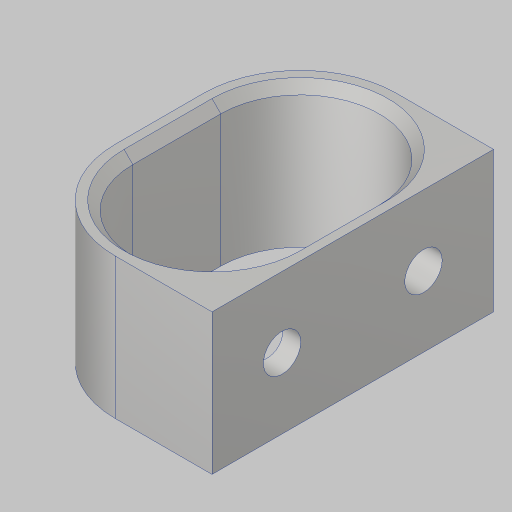
# Autodesk Inventor part: WL-007
Saved by Autodesk Inventor 2023.5 (Build 275446000, 446)
## iProperties
Created: 2025-02-28
Part Number: WL-007
Material: Aluminum 6061
Document SubType Name: Modeling
Designer: slick
Density: 2.7 g/cm^3
Appearance: Aluminum - Flat
Author: slick
Autodesk Inventor part; units mm, degrees
ref_plane "YZ Plane" through (0, 0, 0) normal (1, 0, 0) x (0, 1, 0)
ref_plane "XZ Plane" through (0, 0, 0) normal (0, 1, 0) x (-1, 0, 0)
ref_plane "XY Plane" through (0, 0, 0) normal (0, 0, 1) x (1, 0, 0)
sketch "Sketch1" plane through (0, 0, 0) normal (0, 1, 0) x (-1, 0, 0)
  line L0 (0, -7.9375) -> (0, 7.9375) construction
  line L1 (17.4625, -7.9375) -> (17.4625, 7.9375)
  line L2 (-17.4625, 7.9375) -> (-17.4625, -7.9375)
  arc A0 (-17.4625, -7.9375) -> (17.4625, -7.9375) centre (0, -7.9375) ccw
  arc A1 (17.4625, 7.9375) -> (-17.4625, 7.9375) centre (0, 7.9375) ccw
  line L3 (14.2875, 7.9375) -> (14.2875, -7.9375)
  arc A2 (-14.2875, -7.9375) -> (14.2875, -7.9375) centre (0, -7.9375) ccw
  line L4 (-14.2875, -7.9375) -> (-14.2875, 7.9375)
  arc A3 (14.2875, 7.9375) -> (-14.2875, 7.9375) centre (0, 7.9375) ccw
  point P0 (0, 0)
  point P1 (0, 25.4)
  point P2 (0, -25.4)
  dimension "d1" = 34.925
  dimension "d2" = 3.175
  dimension "d3" = 50.8
  constraints: 12 end point, 10 point on circle, 4 centre point, 4 tangent, 2 parallel, 1 midpoint, 1 vertical, 3 other
  measures "d1" distance between parallel lines of L2 L1
  measures "d2" distance between parallel lines of L1 L3
  measures "d3" distance of point (0, 25.4) point (0, -25.4)
extrude "Extrusion1" add sketch "Sketch1" along normal mid plane 25.4
sketch "Sketch2" plane through (17.4625, -12.7, -7.9375) normal (1, 0, 0) x (0, 0, -1)
  line L0 (0, 0) -> (0, 25.4) construction
  line L1 (-15.875, 25.4) -> (0, 25.4) construction
  line L2 (-15.875, 0) -> (-15.875, 25.4) construction
  line L3 (0, 0) -> (-15.875, 0) construction
  line L4 (-15.875, 0) -> (-15.875, 25.4) construction
  line L5 (-15.875, 25.4) -> (-15.875, 25.4) construction
  line L6 (-15.875, 25.4) -> (-15.875, 0) construction
  line L7 (-15.875, 0) -> (-15.875, 0) construction
  line L8 (0, 0) -> (0, 25.4) construction
  line L9 (0, 25.4) -> (0, 25.4) construction
  line L10 (0, 0) -> (0, 25.4) construction
  line L11 (0, 0) -> (0, 0) construction
  line L12 (-15.875, 25.4) -> (-33.3375, 25.4) construction
  line L13 (17.4625, 0) -> (17.4625, 25.4) construction
  line L14 (-33.3375, 25.4) -> (17.4625, 25.4)
  line L15 (17.4625, 25.4) -> (17.4625, 0)
  line L16 (17.4625, 0) -> (-33.3375, 0)
  line L17 (-33.3375, 0) -> (-33.3375, 25.4)
  line L18 (0, 0) -> (-15.875, 0) construction
  circle A0 centre (-20.701, 12.7) radius 3.375
  circle A1 centre (4.826, 12.7) radius 3.375
  line L19 (-20.701, 12.7) -> (4.826, 12.7) construction
  point P0 (-7.9375, 12.7)
  point P1 (-7.9375, 12.7)
  dimension "d6" = 6.75
  dimension "d7" = 25.527
  constraints: 10 end point, 2 centre point, 2 horizontal, 2 horizontal alignment, 2 parallel, 1 coincident, 1 collinear, 1 equal radius, 1 midpoint, 1 perpendicular, 1 point on line
  measures "d6" diameter of A0
  measures "d7" distance of L19.start L19.end
extrude "Extrusion2" add sketch "Sketch2" against normal up to next
extrude "Extrusion3" cut sketch "Sketch1" along normal mid plane 25.4 contours L3 A2 L4 A3
chamfer "Chamfer1" distance 1.5875 angle 45 4 edges at (-14.2875, 12.7, 0) (0, 12.7, -22.225) (14.2875, 12.7, 0) (0, 12.7, 22.225)
sketch "Sketch3" plane through (17.4625, -12.7, -25.4) normal (1, 0, 0) x (0, 0, -1)
  spline S0 degree 5 poles (-34.7885, 12.7) (-34.7885, 13.1002) (-34.8477, 13.4999) (-34.9664, 13.8945) (-35.1476, 14.2759) (-35.6125, 14.9418) (-35.882, 15.2355) (-36.2063, 15.4983) (-36.5819, 15.7147) (-37.4167, 16.021) (-37.869, 16.1093) (-38.3306, 16.1165) (-38.775, 16.0457) (-39.6369, 15.7746) (-40.0468, 15.5551) (-40.4001, 15.282) (-40.6942, 14.9708) (-41.4114, 13.9437) (-41.6624, 13.1274) (-41.6637, 12.2735) (-41.4107, 11.4552) (-40.6942, 10.4292) (-40.4001, 10.118) (-40.0468, 9.8449) (-39.6369, 9.6254) (-38.775, 9.3543) (-38.3306, 9.2835) (-37.869, 9.2907) (-37.4167, 9.379) (-36.5819, 9.6853) (-36.2063, 9.9017) (-35.882, 10.1645) (-35.6125, 10.4582) (-35.1476, 11.1241) (-34.9664, 11.5055) (-34.8477, 11.9001) (-34.7885, 12.2998) (-34.7885, 12.7) knots 0 0 0 0 0 0 0.105714 0.105714 0.105714 0.105714 0.197568 0.197568 0.197568 0.197568 0.288713 0.288713 0.288713 0.288713 0.393324 0.393324 0.393324 0.393324 0.606047 0.606047 0.606047 0.606047 0.710825 0.710825 0.710825 0.710825 0.802115 0.802115 0.802115 0.802115 0.894116 0.894116 0.894116 0.894116 1 1 1 1 1 1 projected
  spline S1 degree 8 poles (-9.2615, 12.7) (-9.2615, 12.9727) (-9.2867, 13.2451) (-9.337, 13.5153) (-9.4123, 13.7812) (-9.5126, 14.041) (-9.6379, 14.2923) (-9.7881, 14.5328) (-10.13, 14.9766) (-10.3203, 15.1821) (-10.5339, 15.3734) (-10.7705, 15.5476) (-11.0297, 15.7013) (-11.3104, 15.8308) (-11.6111, 15.9319) (-12.1924, 16.0564) (-12.4671, 16.0903) (-12.7489, 16.0984) (-13.033, 16.079) (-13.3141, 16.0321) (-13.587, 15.9588) (-13.8472, 15.8619) (-14.365, 15.6147) (-14.6174, 15.4595) (-14.847, 15.2842) (-15.0532, 15.0927) (-15.2359, 14.8882) (-15.3956, 14.6736) (-15.5324, 14.4518) (-15.8672, 13.7909) (-16.0078, 13.3358) (-16.0746, 12.8709) (-16.0705, 12.4027) (-15.9955, 11.937) (-15.847, 11.4806) (-15.6204, 11.043) (-15.1561, 10.4403) (-14.98, 10.2471) (-14.7818, 10.0645) (-14.562, 9.8963) (-14.3218, 9.7461) (-14.0628, 9.6172) (-13.7871, 9.5131) (-13.2228, 9.3642) (-12.9404, 9.3179) (-12.6543, 9.2993) (-12.3693, 9.3086) (-12.0899, 9.3449) (-11.8204, 9.4062) (-11.5649, 9.4892) (-10.8144, 9.8053) (-10.3703, 10.1058) (-10.0003, 10.4673) (-9.7051, 10.8724) (-9.484, 11.308) (-9.3362, 11.7634) (-9.2615, 12.2302) (-9.2615, 12.7) knots 0 0 0 0 0 0 0 0 0 0.115011 0.115011 0.115011 0.115011 0.115011 0.115011 0.115011 0.224864 0.224864 0.224864 0.224864 0.224864 0.224864 0.224864 0.315487 0.315487 0.315487 0.315487 0.315487 0.315487 0.315487 0.417599 0.417599 0.417599 0.417599 0.417599 0.417599 0.417599 0.613283 0.613283 0.613283 0.613283 0.613283 0.613283 0.613283 0.710373 0.710373 0.710373 0.710373 0.710373 0.710373 0.710373 0.80231 0.80231 0.80231 0.80231 0.80231 0.80231 0.80231 1 1 1 1 1 1 1 1 1 projected
  point P0 (-25.4, 12.7)
  constraints: 2 other
extrude "Extrusion4" cut sketch "Sketch3" against normal blind 6.35
body "Solid1"
